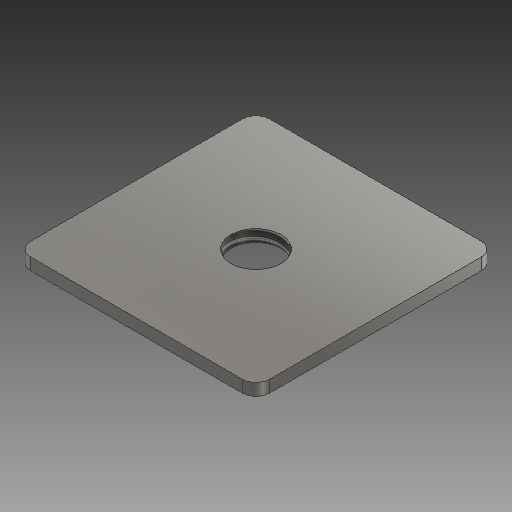
# Autodesk Inventor part: Chapa 40x40
Saved by Autodesk Inventor 2017 (Build 210142000, 142)
## iProperties
Created: 2019-06-15
Part Number: Chapa 40x40
Material: Stainless Steel
Document SubType Name: Sheet Metal
Designer: leonardo.prado
Mass: 24.6488 g
Surface Area: 34.4601 cm^2
Volume: 3.08111 cm^3
Density: 8 g/cm^3
Sheet Metal Rule: Default_mm
Appearance: Semi-Polished
Author: leonardo.prado
Autodesk Inventor part; units mm, degrees
ref_plane "YZ Plane" through (0, 0, 0) normal (1, 0, 0) x (0, 1, 0)
ref_plane "XZ Plane" through (0, 0, 0) normal (0, 1, 0) x (-1, 0, 0)
ref_plane "XY Plane" through (0, 0, 0) normal (0, 0, 1) x (1, 0, 0)
sketch "Sketch1" plane through (0, 0, 0) normal (0, 0, 1) x (1, 0, 0)
  line L0 (17.75, 20) -> (-17.75, 20)
  arc A0 (-17.75, 20) -> (-20, 17.75) centre (-17.75, 17.75) ccw
  line L1 (-20, 17.75) -> (-20, -17.75)
  arc A1 (-20, -17.75) -> (-17.75, -20) centre (-17.75, -17.75) ccw
  line L2 (-17.75, -20) -> (17.75, -20)
  arc A2 (17.75, -20) -> (20, -17.75) centre (17.75, -17.75) ccw
  line L3 (20, -17.75) -> (20, 17.75)
  arc A3 (20, 17.75) -> (17.75, 20) centre (17.75, 17.75) ccw
  point P0 (0, 0)
extrude "Plate1" add sketch "Sketch1" along normal blind 2
sketch "Sketch3" plane through (0, 0, 2) normal (0, 0, 1) x (1, 0, 0)
  point P0 (0, 0)
  point P1 (0, 0)
  constraints: 1 coincident
hole "Hole1" at (0, 0, 2) direction (0, 0, -1) diameter 8.376 depth 2 tip angle 118 thread size "M10x1.5" class "6H" standard "ANSI Metric M Profile"
equation "\"d6\" = Thickness"
equation "\"BendRadius\" = Thickness"
equation "\"BendReliefWidth\" = Thickness"
equation "\"BendReliefDepth\" = 0.5 * Thickness"
equation "\"CornerReliefSize\" = 4 * Thickness"
equation "\"MinimumRemnant\" = 2 * Thickness"
equation "\"TransitionRadius\" = BendRadius"
equation "\"JacobiRadiusSize\" = BendRadius"
equation "\"GapSize\" = Thickness"
equation "\"d0\" = BendRadius"
equation "\"Thickness\" = 2"
body "Solid1"
